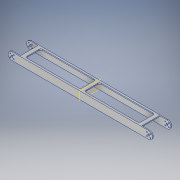
# Autodesk Inventor part: ArmProto2.2Assembly
Saved by Autodesk Inventor 2017 (Build 210142000, 142)
## iProperties
Created: 2017-10-04
Part Number: ArmProto2.2Assembly
Material: Aluminum 6061
Document SubType Name: Modeling
Designer: User
Density: 2.7 g/cm^3
Appearance: Aluminum - Flat
Mass: 245.529 g
Surface Area: 650.625 cm^2
Volume: 90.9365 cm^3
Author: User
Autodesk Inventor part; units mm, degrees
ref_plane "XZ Plane" through (0, 0, 0) normal (0, 1, 0) x (-1, 0, 0)
ref_plane "XY Plane" through (0, 0, 0) normal (0, 0, 1) x (1, 0, 0)
sketch "Sketch1" plane through (0, 0, 0) normal (1, 0, 0) x (0, 1, 0)
  line L0 (0, 0) -> (25.4, 0)
  line L1 (25.4, 0) -> (25.4, -64.6049)
  line L2 (25.4, -64.6049) -> (0, -64.6049)
  line L3 (0, -64.6049) -> (0, 0)
  line L4 (0, -3.175) -> (22.225, -3.175)
  line L5 (22.225, -3.175) -> (22.225, -61.4299)
  line L6 (22.225, -61.4299) -> (0, -61.4299)
  line L7 (0, -61.4299) -> (0, -3.175)
  dimension "d0" = 25.4
  dimension "d2" = 58.2549
  dimension "d3" = 22.225
  dimension "d4" = 3.175
  dimension "d32" = 3.175
  constraints: 16 end point, 4 parallel, 2 horizontal, 2 perpendicular, 1 point on line
  measures "d0" distance of L1.end L2.end
  measures "d2" distance of L4.end L5.end
  measures "d3" distance of L5.end L6.end
  measures "d4" distance between parallel lines of L0 L4
  measures "d32" distance between parallel lines of L6 L2
extrude "Extrusion1" add sketch "Sketch1" along normal blind 482.6 contours L0 L1 L2 L3 L6 L5 L4
sketch "Sketch3" plane through (0, 25.4, 0) normal (0, 1, 0) x (1, 0, 0)
  line L0 (0, 64.6049) -> (0, 0) projected
  line L1 (0, 0) -> (482.6, 0) projected
  line L2 (482.6, 64.6049) -> (482.6, 0) projected
  line L3 (0, 64.6049) -> (482.6, 64.6049) projected
  line L4 (482.6, 3.175) -> (444.5, 3.175)
  line L5 (444.5, 3.175) -> (444.5, 61.4299)
  line L6 (444.5, 61.4299) -> (482.6, 61.4299)
  line L7 (482.6, 61.4299) -> (482.6, 3.175)
  line L8 (0, 64.6049) -> (0, 0) projected
  line L9 (0, 3.175) -> (38.1, 3.175)
  line L10 (38.1, 3.175) -> (38.1, 61.4299)
  line L11 (38.1, 61.4299) -> (0, 61.4299)
  line L12 (0, 61.4299) -> (0, 3.175)
  point P0 (482.6, 61.4299)
  dimension "d14" = 64.6049
  dimension "d16" = 38.1
  dimension "d27" = 38.1
  dimension "d28" = 58.2549
  dimension "d29" = 3.175
  dimension "d30" = 58.2549
  dimension "d31" = 3.175
  constraints: 16 end point, 4 parallel, 2 horizontal, 2 perpendicular, 2 point on line
  measures "d14" distance of L0.start L0.end
  measures "d16" distance of L5.end L6.end
  measures "d27" distance of L11.end L10.end
  measures "d28" distance of L9.end L10.end
  measures "d29" distance between parallel lines of L3 L11
  measures "d30" distance of L4.end L5.end
  measures "d31" distance between parallel lines of L3 L6
extrude "Extrusion2" cut sketch "Sketch3" against normal blind 3.175 contours L11 L10 L9 L0 | L2 L4 L5 L6
sketch "Sketch4" plane through (0, 0, 0) normal (0, 0, 1) x (1, 0, 0)
  line L0 (0, 25.4) -> (0, 0) projected
  line L1 (0, 0) -> (482.6, 0) projected
  line L2 (482.6, 25.4) -> (482.6, 0) projected
  line L3 (0, 25.4) -> (482.6, 25.4) projected
  circle A0 centre (12.7, 12.7) radius 3.175
  circle A1 centre (469.9, 12.7) radius 3.175
  line L4 (7.0485, 18.3515) -> (18.3515, 18.3515)
  line L5 (18.3515, 18.3515) -> (18.3515, 7.0485)
  line L6 (18.3515, 7.0485) -> (7.0485, 7.0485)
  line L7 (7.0485, 7.0485) -> (7.0485, 18.3515)
  line L8 (464.2485, 18.3515) -> (475.5515, 18.3515)
  line L9 (475.5515, 18.3515) -> (475.5515, 7.0485)
  line L10 (475.5515, 7.0485) -> (464.2485, 7.0485)
  line L11 (464.2485, 7.0485) -> (464.2485, 18.3515)
  dimension "d19" = 6.35
  dimension "d20" = 12.7
  dimension "d21" = 25.4
  dimension "d22" = 12.7
  dimension "d23" = 6.35
  dimension "d24" = 12.7
  dimension "d33" = 11.303
  dimension "d34" = 11.303
  dimension "d35" = 7.0485
  dimension "d36" = 7.0485
  dimension "d37" = 11.303
  dimension "d38" = 11.303
  dimension "d39" = 7.0485
  dimension "d40" = 7.0485
  constraints: 16 end point, 8 coincident, 4 parallel, 2 centre point, 2 horizontal, 2 perpendicular
  measures "d19" diameter of A0
  measures "d20" distance from line of L0 A0.centre
  measures "d21" distance of L0.start L0.end
  measures "d22" distance from line of L1 A0.centre
  measures "d23" diameter of A1
  measures "d24" distance from line of L2 A1.centre
  measures "d33" distance of L5.end L6.end
  measures "d34" distance of L4.end L5.end
  measures "d35" distance between parallel lines of L3 L4
  measures "d36" distance between parallel lines of L0 L7
  measures "d37" distance of L9.end L10.end
  measures "d38" distance of L8.end L9.end
  measures "d39" distance between parallel lines of L3 L8
  measures "d40" distance between parallel lines of L2 L9
extrude "Extrusion3" cut sketch "Sketch4" against normal blind 127 contours A0 | A1
sketch "Sketch5" plane through (0, 0, 0) normal (0, 0, 1) x (1, 0, 0)
  line L0 (-0.0027, 25.404) -> (-0.0027, -0.0046)
  line L1 (-0.0027, -0.0046) -> (482.6, -0.0046)
  line L2 (-0.0027, 25.404) -> (482.6, 25.404)
  line L3 (7.0501, 18.3512) -> (18.3531, 18.3512)
  line L4 (18.3531, 18.3512) -> (18.3531, 7.0482)
  line L5 (18.3531, 7.0482) -> (7.0501, 7.0482)
  line L6 (7.0501, 7.0482) -> (7.0501, 18.3512)
  line L7 (464.2442, 18.3512) -> (475.5472, 18.3512)
  line L8 (475.5472, 18.3512) -> (475.5472, 7.0482)
  line L9 (475.5472, 7.0482) -> (464.2442, 7.0482)
  line L10 (464.2442, 7.0482) -> (464.2442, 18.3512)
  line L11 (482.6, 25.4) -> (482.6, 0) projected
  point P0 (0, 0)
  point P1 (0, 0)
  dimension "d43" = 25.4086
  dimension "d47" = 11.303
  dimension "d48" = 11.303
  dimension "d49" = 7.0528
  dimension "d50" = 7.0528
  dimension "d51" = 11.303
  dimension "d52" = 11.303
  dimension "d53" = 7.0528
  dimension "d63" = 18.3558
  constraints: 22 end point, 8 coincident, 4 parallel, 2 horizontal, 2 perpendicular, 2 point on line
  measures "d43" distance of L0.start L0.end
  measures "d47" distance of L4.end L5.end
  measures "d48" distance of L3.end L4.end
  measures "d49" distance between parallel lines of L2 L3
  measures "d50" distance between parallel lines of L0 L6
  measures "d51" distance of L8.end L9.end
  measures "d52" distance of L7.end L8.end
  measures "d53" distance between parallel lines of L2 L7
  measures "d63" distance between parallel lines of L10 L11
hole "Hole1" at (7.0501, 18.3512, 0) at (18.3531, 18.3512, 0) at (18.3531, 7.0482, 0) at (7.0501, 7.0482, 0) at (464.2442, 18.3512, 0) at (475.5472, 18.3512, 0) at (475.5472, 7.0482, 0) at (464.2442, 7.0482, 0) direction (0, 0, -1) diameter 3.5 depth 127 tip angle 118
fillet "Fillet1" radius 12.7 8 edges at (482.6, 25.4, -1.5875) (482.6, 0, -1.5875) (482.6, 25.4, -63.0174) (482.6, 0, -63.0174) (0, 25.4, -1.5875) (0, 0, -1.5875) (0, 0, -63.0174) (0, 25.4, -63.0174)
sketch "Sketch6" plane through (38.1, 25.4, -3.175) normal (0, 1, 0) x (1, 0, 0)
  line L0 (-25.4, 58.2549) -> (-25.4, 61.4299) projected
  line L1 (-25.4, 58.2549) -> (0, 58.2549) projected
  line L2 (0, 58.2549) -> (0, 0) projected
  line L3 (0, 0) -> (-25.4, 0) projected
  line L4 (-25.4, -3.175) -> (-25.4, 0) projected
  line L5 (-25.4, -3.175) -> (431.8, -3.175) projected
  line L6 (431.8, 0) -> (431.8, -3.175) projected
  line L7 (431.8, 0) -> (406.4, 0) projected
  line L8 (406.4, 0) -> (406.4, 58.2549) projected
  line L9 (406.4, 58.2549) -> (431.8, 58.2549) projected
  line L10 (431.8, 61.4299) -> (431.8, 58.2549) projected
  line L11 (-25.4, 61.4299) -> (431.8, 61.4299) projected
  line L12 (12.7, 55.0799) -> (196.85, 55.0799)
  line L13 (196.85, 55.0799) -> (196.85, 3.175)
  line L14 (196.85, 3.175) -> (12.7, 3.175)
  line L15 (12.7, 3.175) -> (12.7, 55.0799)
  point P0 (-38.1, -3.175)
  dimension "d65" = 406.4
  dimension "d66" = 64.6049
  dimension "d67" = 6.35
  dimension "d68" = 51.9049
  dimension "d69" = 12.7
  dimension "d70" = 184.15
  constraints: 8 end point, 2 parallel, 1 horizontal, 1 perpendicular
  measures "d65" distance between parallel lines of L8 L2
  measures "d66" distance between parallel lines of L5 L11
  measures "d67" distance between parallel lines of L11 L12
  measures "d68" distance of L14.end L12.start
  measures "d69" distance between parallel lines of L2 L15
  measures "d70" distance of L12.start L12.end
extrude "Extrusion4" cut sketch "Sketch6" against normal blind 25.4 contours L12 L13 L14 L15
fillet "Fillet2" radius 6.35 4 edges at (234.95, 23.8125, -58.2549) (234.95, 23.8125, -6.35) (50.8, 23.8125, -6.35) (50.8, 23.8125, -58.2549)
ref_plane "Work Plane1" through (241.3, 25.4, -64.6049) normal (1, 0, 0) x (0, 1, 0)
mirror "Mirror1" about plane through (241.3, 25.4, -64.6049) normal (1, 0, 0) of "Extrusion4"
fillet "Fillet3" radius 6.35 4 edges at (247.65, 23.8125, -6.35) (247.65, 23.8125, -58.2549) (431.8, 23.8125, -58.2549) (431.8, 23.8125, -6.35)
equation "\"d32\" = d4"
equation "\"d30\" = d28"
equation "\"d31\" = d29"
equation "\"d22\" = 0.5 * d21"
equation "\"d23\" = d19"
equation "\"d24\" = d20"
equation "\"d35\" = -0.5 * d34 + 0.5 * d21"
equation "\"d36\" = d35"
equation "\"d37\" = d33"
equation "\"d38\" = d34"
equation "\"d39\" = d35"
equation "\"d40\" = d36"
equation "\"d49\" = -0.5 * d48 + 0.5 * d43"
equation "\"d50\" = d49"
equation "\"d51\" = d47"
equation "\"d52\" = d48"
equation "\"d53\" = d49"
equation "\"d63\" = d51 + d50"
body "Solid1"
